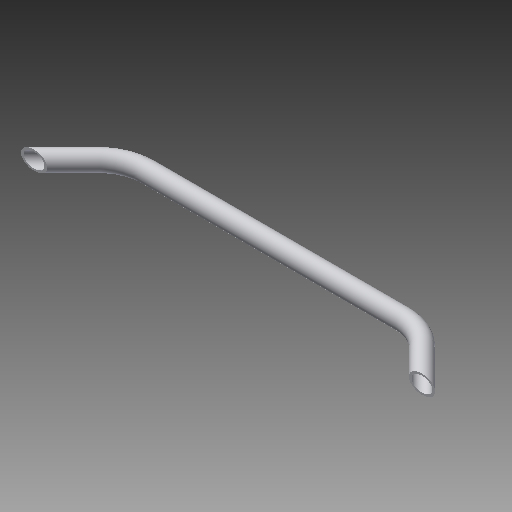
# Autodesk Inventor part: Rura_barierka_oparcia
Saved by Autodesk Inventor 2017 (Build 210142000, 142)
## iProperties
Created: 2015-11-22
Part Number: Rura_barierka_oparcia
Material: Aluminium AW-7020
Document SubType Name: Modelowanie
Designer: graaapsik
Density: 2.78 g/cm^3
Appearance: Aluminium AW-7020
Sheet Metal Rule: Default_mm
Mass: 143.057 g
Surface Area: 517.792 cm^2
Volume: 51.4593 cm^3
Author: graaapsik
Autodesk Inventor part; units mm, degrees
note: some values were not read from the file. Chosen so that the rebuilt part matches the saved one: bend side of "Gięcie części2".
ref_plane "YZ Plane" through (0, 0, 0) normal (1, 0, 0) x (0, 1, 0)
ref_plane "XZ Plane" through (0, 0, 0) normal (0, 1, 0) x (-1, 0, 0)
ref_plane "XY Plane" through (0, 0, 0) normal (0, 0, 1) x (1, 0, 0)
sketch "Szkic1" plane through (0, 0, 0) normal (1, 0, 0) x (0, 1, 0)
  circle A0 centre (0, 0) radius 10
  dimension "d0" = 20
  constraints: 1 centre point, 1 coincident
  measures "d0" diameter of A0
extrude "Wyciągnięcie proste1" add sketch "Szkic1" along normal blind 475
shell "Skorupa1" thickness 2 removed faces 2 at (475, -1.182, 3.1167) at (0, -1.182, 3.1167)
sketch "Szkic2" plane through (0, 0, 0) normal (0, 0, 1) x (1, 0, 0)
  line L0 (100, 28.3712) -> (100, -25.6691)
  line L1 (0, 10) -> (0, -10) projected
  point P0 (0, 0)
  dimension "d4" = 100
  constraints: 2 end point, 1 vertical
  measures "d4" distance between parallel lines of L1 L0
bend part "Gięcie części1" radius 50.9296 angle 45 line through (100, 28.3712, 0) along (0, -1, 0) centre toward (0, 0, 1) moving side (-1, 0, 0) both sides no
sketch "Szkic3" plane through (0, 0, 0) normal (0, 0, 1) x (1, 0, 0)
  line L0 (375, 37.2706) -> (375, -31.4113)
  line L1 (475, -10) -> (475, 10) projected
  point P0 (0, 0)
  dimension "d7" = 100
  constraints: 2 end point, 1 vertical
  measures "d7" distance between parallel lines of L0 L1
bend part "Gięcie części2" radius 50.9296 angle 45 line through (375, 37.2706, 0) along (0, -1, 0) centre toward (0, 0, 1) moving side (1, 0, 0) both sides no
sketch "Szkic4" plane through (0, 0, 0) normal (0, 1, 0) x (-1, 0, 0)
  line L0 (-446.368, 64.4144) -> (-460.5101, 50.2723) construction
  line L1 (-403.9416, 21.988) -> (-446.368, 64.4144) construction
  line L2 (-418.0837, 7.8459) -> (-460.5101, 50.2723) construction
  line L3 (-460.5101, 50.2723) -> (-446.368, 64.4144)
  line L4 (-446.368, 64.4144) -> (-432.2259, 50.2723)
  line L5 (-432.2259, 50.2723) -> (-460.5101, 50.2723)
  line L6 (-14.4899, 50.2723) -> (-28.632, 64.4144) construction
  line L7 (-28.632, 64.4144) -> (-71.0584, 21.988) construction
  line L8 (-14.4899, 50.2723) -> (-56.9163, 7.8459) construction
  line L9 (-14.4899, 50.2723) -> (-28.632, 64.4144)
  line L10 (-28.632, 64.4144) -> (-42.7741, 50.2723)
  line L11 (-42.7741, 50.2723) -> (-14.4899, 50.2723)
  point P0 (0, 0)
  constraints: 12 end point, 2 collinear, 2 point on line, 1 horizontal, 1 perpendicular
extrude "Wyciągnięcie proste2" cut sketch "Szkic4" along normal mid plane 20
equation "\"PromieńGięcia\" = Grubość"
equation "\"SzerokośćGięciaPodcięcia\" = Grubość"
equation "\"GłębokośćGięciaPodcięcia\" = 0.5 * Grubość"
equation "\"RozmiarPodcięciaNarożnika\" = 4 * Grubość"
equation "\"MinimalnaPozostałość\" = 2 * Grubość"
equation "\"PromieńPrzejścia\" = PromieńGięcia"
equation "\"Rozmiar_promienia_Jacobiego\" = PromieńGięcia"
equation "\"Wielk_odstępu\" = Grubość"
equation "\"Grubość\" = 0.5"
